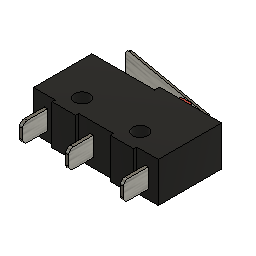
limit switch - small v3 (Autodesk Fusion 360 design; units mm, degrees)
Autodesk Fusion 360 part; units mm, degrees
sketch "Sketch1" plane through (0, 0, 0) normal (0, 1, 0) x (1, 0, 0)
  line L0 (0, 0) -> (0, -9.42)
  line L1 (0, -9.42) -> (3.47, -9.42)
  line L2 (3.47, -9.42) -> (3.47, -9.92)
  line L3 (3.47, -9.92) -> (7.27, -9.92)
  line L4 (7.27, -9.92) -> (7.27, -9.42)
  line L5 (7.27, -9.42) -> (12.87, -9.42)
  line L6 (12.87, -9.42) -> (12.87, -9.92)
  line L7 (12.87, -9.92) -> (16.67, -9.92)
  line L8 (20.14, 0.8) -> (10.125, 0.8)
  line L9 (10.125, 0.8) -> (10.125, 0)
  line L10 (10.125, 0) -> (0, 0)
  circle A0 centre (5.37, -6.97) radius 1.2
  circle A1 centre (14.77, -6.97) radius 1.2
  line L11 (16.67, -9.92) -> (16.67, -9.42)
  line L12 (16.67, -9.42) -> (20.14, -9.42)
  line L13 (20.14, -9.42) -> (20.14, 0.8)
  line L14 (12.04, 0.8) -> (12.04, 1.8)
  line L15 (12.54, 2.3) -> (13.54, 2.3)
  line L16 (14.04, 1.8) -> (14.04, 0.8)
  line L17 (16.915, 0.8) -> (16.915, 2.1)
  line L18 (16.915, 2.1) -> (0.9116, 4.9201)
  line L19 (0.9116, 4.9201) -> (0.8552, 4.6)
  line L20 (0.8552, 4.6) -> (16.59, 1.8273)
  line L21 (16.59, 1.8273) -> (16.59, 0.8)
  line L22 (1.75, -9.42) -> (1.75, -13.42)
  line L23 (1.75, -13.42) -> (2.25, -13.42)
  line L24 (2.25, -13.42) -> (2.25, -9.42)
  line L25 (9.17, -9.42) -> (9.17, -13.42)
  line L26 (9.17, -13.42) -> (9.67, -13.42)
  line L27 (9.67, -13.42) -> (9.67, -9.42)
  line L28 (18.01, -9.42) -> (18.01, -13.42)
  line L29 (18.01, -13.42) -> (18.51, -13.42)
  line L30 (18.51, -13.42) -> (18.51, -9.42)
  arc A2 (12.54, 2.3) -> (12.04, 1.8) centre (12.54, 1.8) ccw
  arc A3 (14.04, 1.8) -> (13.54, 2.3) centre (13.54, 1.8) ccw
  line L31 (5.37, -9.92) -> (5.37, -6.97) construction
  line L32 (14.77, -9.92) -> (14.77, -6.97) construction
  line L33 (5.37, -6.97) -> (14.77, -6.97) construction
  dimension "d3" = 9.42
  dimension "d4" = 9.92
  dimension "d5" = 4
  dimension "d6" = 0.5
  dimension "d7" = 0.5
  dimension "d8" = 0.5
  dimension "d9" = 9.34
  dimension "d10" = 7.92
  dimension "d11" = 1.75
  dimension "d12" = 3.47
  dimension "d13" = 3.47
  dimension "d14" = 5.6
  dimension "d15" = 3.8
  dimension "d16" = 3.8
  dimension "d17" = 19.8
  dimension "d18" = 0.8
  dimension "d19" = 10.015
  dimension "d20" = 3.225
  dimension "d22" = 6.1
  dimension "d23" = 2
  dimension "d24" = 1.5
  dimension "d25" = 0.325
  dimension "d26" = 0.325
  dimension "d27" = 1.3
  dimension "d28" = 16.25
  dimension "d29" = 0.5
  dimension "d30" = 0.5
  dimension "d31" = 4.6
  dimension "d32" = 2.4
  dimension "d33" = 1.75
  constraint coincident L0.start L10.end
  constraint vertical L0
  constraint perpendicular L0 L1
  constraint perpendicular L1 L2
  constraint perpendicular L2 L3
  constraint perpendicular L3 L4
  constraint perpendicular L4 L5
  constraint perpendicular L3 L6
  constraint perpendicular L6 L7
  constraint perpendicular L7 L11
  constraint perpendicular L12 L13
  constraint coincident L8 L14.start
  constraint perpendicular L14 L15
  constraint coincident L8 L16.end
  constraint coincident L8 L17.start
  constraint perpendicular L18 L19
  constraint perpendicular L19 L20
  constraint coincident L8 L21.end
  constraint coincident L1 L22.start
  constraint perpendicular L1 L22
  constraint perpendicular L17 L23
  constraint perpendicular L1 L24
  constraint coincident L5 L25.start
  constraint perpendicular L5 L25
  constraint perpendicular L2 L26
  constraint perpendicular L5 L27
  constraint perpendicular L28 L29
  constraint coincident L12 L30.end
  constraint perpendicular L12 L30
  constraint parallel L0 L13
  constraint parallel L1 L10
  constraint perpendicular L8 L13
  constraint collinear L1 L5
  constraint collinear L5 L12
  constraint collinear L3 L7
  constraint coincident L12 L28.start
  constraint coincident L5 L27.end
  constraint coincident L1 L24.end
  constraint perpendicular L23 L24
  constraint collinear L23 L26
  constraint collinear L26 L29
  constraint equal A0 A1
  constraint perpendicular L8 L9
  constraint parallel L13 L21
  constraint parallel L16 L21
  constraint parallel L14 L16
  constraint tangent L14 A2
  constraint tangent L15 A2
  constraint tangent L15 A3
  constraint tangent L16 A3
  constraint midpoint L3 L31.start
  constraint coincident A0.centre L31.end
  constraint midpoint L7 L32.start
  constraint coincident A1.centre L32.end
  constraint perpendicular L7 L32
  constraint perpendicular L3 L31
  constraint perpendicular L32 L33
  measures "d3" distance of L1 L10
  measures "d4" distance of L3 L10
  measures "d5" distance of L1 L23
  measures "d6" distance of L22 L24
  measures "d7" distance of L25 L27
  measures "d8" distance of L28 L30 L1.end
  measures "d9" distance of L25 L30
  measures "d10" distance of L22 L27
  measures "d11" distance of L0 L22
  measures "d12" distance of L0 L2
  measures "d13" distance of L11 L13
  measures "d14" distance of L4 L6
  measures "d15" distance of L2 L4
  measures "d16" distance of L6 L11
  measures "d18" distance of L8 L10
  measures "d19" distance of L9 L13
  measures "d20" distance of L13 L17
  measures "d22" distance of L13 L16
  measures "d23" distance of L14 L16
  measures "d24" distance of L8 L15
  measures "d25" distance of L18 L20
  measures "d26" distance of L17 L21
  measures "d27" distance of L8 L17.end
  measures "d28" distance of L17.end L18.end
  measures "d29" radius of A2
  measures "d30" radius of A3
  measures "d31" distance of L10 L19.end
  measures "d32" diameter of A0
  measures "d33" distance of L3 A0
extrude "Extrude1" add sketch "Sketch1" along normal blind 6.45 contours L0 L1 L2 L3 L4 L5 L6 L7 L8 L9 L10 L11 L12 L13 makes body 1
extrude "Extrude2" add sketch "Sketch1" along normal blind 3.1 from surface at 1.5 contours L1 L22 L23 L24 | L5 L25 L26 L27 | L12 L28 L29 L30 bodies 1
extrude "Extrude3" add sketch "Sketch1" along normal blind 4 from surface at 1.3 contours L8 L14 L15 L16 A2 A3 | L8 L17 L18 L19 L20 L21 bodies 1
fillet "Fillet1" radius 0.75 8 edges at (0.8834, 5.3, -4.76) (0.8834, 1.3, -4.76) (2, 4.6, 13.42) (2, 1.5, 13.42) (9.42, 4.6, 13.42) (9.42, 1.5, 13.42) (18.26, 4.6, 13.42) (18.26, 1.5, 13.42) on bodies 1
split "Split1" by plane through (12.04, 0, -0.8) normal (0, 0, -1) bodies 1 makes body 2 at (12.8733, 2.6333, -2.3) makes body 3 at (11.8267, 2.6333, -2.9966)
copy_body "Body->Comp1" bodies 2 removing the originals makes body 4 in component "Button"
copy_body "Body->Comp2" bodies 3 removing the originals makes body 5 in component "Lever"
sketch "Sketch2" plane through (0, 0, -0.8) normal (0, 0, -1) x (-1, 0, 0)
  line L0 (-20.14, 0) -> (-10.125, 0)
  line L1 (-10.125, 0) -> (-10.125, 6.45)
  line L2 (-10.125, 6.45) -> (-20.14, 6.45)
  line L3 (-20.14, 6.45) -> (-20.14, 0)
  line L4 (-14.04, 1.3) -> (-14.04, 5.3) construction
  line L5 (-14.04, 5.3) -> (-12.04, 5.3) construction
  line L6 (-12.04, 5.3) -> (-12.04, 1.3) construction
  line L7 (-12.04, 1.3) -> (-14.04, 1.3) construction
  line L8 (-12.04, 3.3) -> (-14.04, 3.3) construction
  line L9 (-13.04, 5.3) -> (-13.04, 1.3) construction
  line L10 (-16.915, 5.3) -> (-16.59, 5.3)
  line L11 (-16.59, 5.3) -> (-16.59, 1.3)
  line L12 (-16.59, 1.3) -> (-16.915, 1.3)
  line L13 (-16.915, 1.3) -> (-16.915, 5.3)
  line L14 (-16.7525, 1.3) -> (-16.7525, 5.3) construction
  point P0 (-13.04, 3.3)
  constraint midpoint L6 L8.start
  constraint midpoint L4 L8.end
  constraint midpoint L5 L9.start
  constraint midpoint L7 L9.end
  constraint midpoint L9 P0
  constraint midpoint L12 L14.start
  constraint midpoint L10 L14.end
sketch "Sketch3" plane through (0, 1.3, 0) normal (0, -1, 0) x (1, 0, 0)
  line L0 (1.5938, -4.4698) -> (1.6502, -4.7899)
  line L1 (1.6502, -4.7899) -> (16.915, -2.1)
  line L2 (16.915, -2.1) -> (16.915, -0.8)
  line L3 (16.915, -0.8) -> (16.59, -0.8)
  line L4 (16.59, -0.8) -> (16.59, -1.8273)
  line L5 (16.59, -1.8273) -> (1.5938, -4.4698)
component "Button" placed x (1, 0, 0) y (0, 1, 0) z (0, 0, 1) at (0, 0, 0)
component "Lever" placed x (1, 0, 0) y (0, 1, 0) z (0, 0, 1) at (0, 0, 0)
equation "d7 = d6"
equation "d8 = d6"
equation "d13 = d12"
equation "d16 = d15"
equation "d26 = d25"
equation "d30 = d29"
